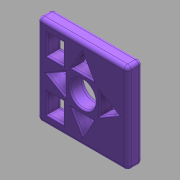
# Autodesk Inventor part: Vo_Nut_Bam
Saved by Autodesk Inventor 2016 (Build 200138000, 138)
## iProperties
Created: 2016-08-15
Part Number: Vo_Nut_Bam
Material: Water
Document SubType Name: Modeling
Designer: ADMIN
Density: 0.9983 g/cm^3
Appearance: Violet
Author: ADMIN
Autodesk Inventor part; units mm, degrees
ref_plane "YZ Plane" through (0, 0, 0) normal (1, 0, 0) x (0, 1, 0)
ref_plane "XZ Plane" through (0, 0, 0) normal (0, 1, 0) x (-1, 0, 0)
ref_plane "XY Plane" through (0, 0, 0) normal (0, 0, 1) x (1, 0, 0)
sketch "Sketch1" plane through (0, 0, 0) normal (0, 1, 0) x (-1, 0, 0)
  circle A0 centre (0, 0) radius 15
  line L0 (0, -25) -> (10.866, -25)
  line L1 (0, -25) -> (-10.866, -25)
  line L2 (-10.866, -25) -> (0, -43.8205)
  line L3 (0, -43.8205) -> (10.866, -25)
  circle A1 centre (0, 0) radius 16.5
  line L4 (13.4641, -23.5) -> (0, -23.5)
  line L5 (0, -23.5) -> (-13.4641, -23.5)
  line L6 (-13.4641, -23.5) -> (0, -46.8205)
  line L7 (0, -46.8205) -> (13.4641, -23.5)
  line L8 (25, 0) -> (25, 10.866)
  line L9 (25, 0) -> (25, -10.866)
  line L10 (25, -10.866) -> (43.8205, 0)
  line L11 (43.8205, 0) -> (25, 10.866)
  line L12 (23.5, 13.4641) -> (23.5, 0)
  line L13 (23.5, 0) -> (23.5, -13.4641)
  line L14 (23.5, -13.4641) -> (46.8205, 0)
  line L15 (46.8205, 0) -> (23.5, 13.4641)
  line L16 (0, 25) -> (-10.866, 25)
  line L17 (0, 25) -> (10.866, 25)
  line L18 (10.866, 25) -> (0, 43.8205)
  line L19 (0, 43.8205) -> (-10.866, 25)
  line L20 (-13.4641, 23.5) -> (0, 23.5)
  line L21 (0, 23.5) -> (13.4641, 23.5)
  line L22 (13.4641, 23.5) -> (0, 46.8205)
  line L23 (0, 46.8205) -> (-13.4641, 23.5)
  line L24 (-25, 0) -> (-25, -10.866)
  line L25 (-25, 0) -> (-25, 10.866)
  line L26 (-25, 10.866) -> (-43.8205, 0)
  line L27 (-43.8205, 0) -> (-25, -10.866)
  line L28 (-23.5, -13.4641) -> (-23.5, 0)
  line L29 (-23.5, 0) -> (-23.5, 13.4641)
  line L30 (-23.5, 13.4641) -> (-46.8205, 0)
  line L31 (-46.8205, 0) -> (-23.5, -13.4641)
  line L32 (46.8205, 46.8205) -> (25.8205, 46.8205)
  line L33 (25.8205, 46.8205) -> (25.8205, 20.8205)
  line L34 (25.8205, 20.8205) -> (46.8205, 20.8205)
  line L35 (46.8205, 20.8205) -> (46.8205, 46.8205)
  line L36 (46.8205, -46.8205) -> (25.8205, -46.8205)
  line L37 (25.8205, -46.8205) -> (25.8205, -20.8205)
  line L38 (25.8205, -20.8205) -> (46.8205, -20.8205)
  line L39 (46.8205, -20.8205) -> (46.8205, -46.8205)
  line L40 (27.3205, 22.3205) -> (27.3205, 45.3205)
  line L41 (27.3205, 45.3205) -> (45.3205, 45.3205)
  line L42 (45.3205, 45.3205) -> (45.3205, 22.3205)
  line L43 (45.3205, 22.3205) -> (27.3205, 22.3205)
  line L44 (45.3205, -45.3205) -> (27.3205, -45.3205)
  line L45 (27.3205, -45.3205) -> (27.3205, -22.3205)
  line L46 (27.3205, -22.3205) -> (45.3205, -22.3205)
  line L47 (45.3205, -22.3205) -> (45.3205, -45.3205)
  line L48 (0, 60) -> (60, 60)
  line L49 (60, 60) -> (60, -60)
  line L50 (60, -60) -> (-60, -60)
  line L51 (-60, -60) -> (-60, 60)
  line L52 (-60, 60) -> (0, 60)
  dimension "d0" = 30
  dimension "d5" = 33
  dimension "d6" = 1.5
  dimension "d10" = 360
  dimension "d12" = 21
  dimension "d13" = 26
  dimension "d14" = 21
  dimension "d15" = 26
  dimension "d16" = 1.5
  dimension "d17" = 1.5
  dimension "d18" = 60
  dimension "d19" = 120
  dimension "d20" = 120
  dimension "d21" = 120
  constraints: 106 end point, 8 parallel, 6 perpendicular, 5 horizontal, 2 centre point, 2 coincident, 1 point on line, 74 other
  measures "d0" diameter of A0
  measures "d5" diameter of A1
  measures "d6" distance between parallel lines of L0 L4
  measures "d12" distance of L34.end L33.end
  measures "d13" distance of L33.end L32.end
  measures "d14" distance of L37.end L38.end
  measures "d15" distance of L36.end L37.end
  measures "d16" distance between parallel lines of L33 L40
  measures "d17" distance between parallel lines of L39 L47
  measures "d18" distance of L48.start L48.end
  measures "d19" distance of L48.end L49.end
  measures "d20" distance of L49.end L50.end
  measures "d21" distance of L50.end L51.end
extrude "Extrusion1" add sketch "Sketch1" along normal blind 20 contours L48 L49 L50 L51 L52
sketch "Sketch2" plane through (0, 20, 0) normal (0, 1, 0) x (1, 0, 0)
  line L0 (-49.5, -21) -> (-49.5, -49.3205)
  line L1 (-49.5, -49.3205) -> (-23.5, -49.3205)
  line L2 (-23.5, -49.3205) -> (-23.5, -18.3205)
  line L3 (-23.5, -18.3205) -> (-49.5, -18.3205)
  line L4 (-49.5, -18.3205) -> (-49.5, -49.3205)
  line L5 (-49.5, 21) -> (-49.5, 49.3205)
  line L6 (-49.5, 49.3205) -> (-23.5, 49.3205)
  line L7 (-23.5, 49.3205) -> (-23.5, 18.3205)
  line L8 (-23.5, 18.3205) -> (-49.5, 18.3205)
  line L9 (-49.5, 18.3205) -> (-49.5, 49.3205)
  line L10 (-21, 0) -> (-21, 17.7942)
  line L11 (-51.8205, 0) -> (-21, 17.7942)
  line L12 (-21, -17.7942) -> (-51.8205, 0)
  line L13 (-21, 0) -> (-21, -17.7942)
  line L14 (0, -21) -> (-17.7942, -21)
  line L15 (0, -51.8205) -> (-17.7942, -21)
  line L16 (17.7942, -21) -> (0, -51.8205)
  line L17 (0, -21) -> (17.7942, -21)
  line L18 (21, 0) -> (21, -17.7942)
  line L19 (51.8205, 0) -> (21, -17.7942)
  line L20 (21, 17.7942) -> (51.8205, 0)
  line L21 (21, 0) -> (21, 17.7942)
  line L22 (0, 21) -> (17.7942, 21)
  line L23 (0, 51.8205) -> (17.7942, 21)
  line L24 (-17.7942, 21) -> (0, 51.8205)
  line L25 (0, 21) -> (-17.7942, 21)
  circle A0 centre (0, 0) radius 19
  point P0 (-25.8205, -46.8205)
  point P1 (-25.8205, 46.8205)
  dimension "d34" = 360
  constraints: 52 end point, 2 parallel, 2 vertical, 1 centre point, 1 coincident, 1 horizontal, 1 perpendicular, 33 other
extrude "Extrusion2" cut sketch "Sketch2" against normal blind 4
fillet "Fillet1" radius 5 4 edges at (-60, 10, -60) (60, 10, -60) (60, 10, 60) (-60, 10, 60)
fillet "Fillet2" radius 5 8 edges at (-58.5355, 0, 58.5355) (-60, 0, 0) (-58.5355, 0, -58.5355) (0, 0, -60) (58.5355, 0, -58.5355) (60, 0, 0) (58.5355, 0, 58.5355) (0, 0, 60)
fillet "Fillet3" radius 2 21 edges at (-35.1603, 0, 6.7321) (-35.1603, 0, -6.7321) (-23.5, 0, 0) (-25.8205, 0, -33.8205) (-36.3205, 0, -20.8205) (-46.8205, 0, -33.8205) (-36.3205, 0, -46.8205) (6.7321, 0, -35.1603) (-6.7321, 0, -35.1603) (0, 0, -23.5) (35.1603, 0, -6.7321) (23.5, 0, 0) (35.1603, 0, 6.7321) (16.5, 0, 0) (0, 0, 23.5) (6.7321, 0, 35.1603) (-6.7321, 0, 35.1603) (-25.8205, 0, 33.8205) (-36.3205, 0, 20.8205) (-46.8205, 0, 33.8205) (-36.3205, 0, 46.8205)
fillet "Fillet4" radius 5 8 edges at (-58.5355, 20, 58.5355) (0, 20, 60) (58.5355, 20, 58.5355) (60, 20, 0) (58.5355, 20, -58.5355) (0, 20, -60) (-58.5355, 20, -58.5355) (-60, 20, 0)
fillet "Fillet5" radius 1 18 edges at (16.5, 16, 0) (-25.8205, 16, 33.8205) (-36.3205, 16, 46.8205) (-46.8205, 16, 33.8205) (-36.3205, 16, 20.8205) (-36.3205, 16, -20.8205) (-46.8205, 16, -33.8205) (-25.8205, 16, -33.8205) (-36.3205, 16, -46.8205) (0, 16, -23.5) (-6.7321, 16, -35.1603) (6.7321, 16, -35.1603) (6.7321, 16, 35.1603) (-6.7321, 16, 35.1603) (0, 16, 23.5) (35.1603, 16, 6.7321) (23.5, 16, 0) (35.1603, 16, -6.7321)
body "Solid1"
